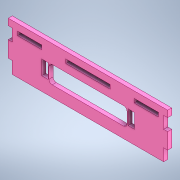
# Autodesk Inventor part: case top back
Saved by Autodesk Inventor 2022.3 (Build 263350030, 350C)
## iProperties
Created: 2021-05-28
Part Number: case top back
Material: Lead
Document SubType Name: Modeling
Designer: benka
Density: 11.34 g/cm^3
Appearance: Pink
Mass: 464.918 g
Surface Area: 220.363 cm^2
Volume: 40.9981 cm^3
Author: benka
Autodesk Inventor part; units mm, degrees
ref_plane "YZ Plane" through (0, 0, 0) normal (1, 0, 0) x (0, 1, 0)
ref_plane "XZ Plane" through (0, 0, 0) normal (0, 1, 0) x (-1, 0, 0)
ref_plane "XY Plane" through (0, 0, 0) normal (0, 0, 1) x (1, 0, 0)
sketch "Sketch1" plane through (0, 0, 0) normal (0, 0, 1) x (1, 0, 0)
  line L0 (49.9396, 9.6174) -> (57.9396, 9.6174)
  line L1 (57.9396, -8.4526) -> (49.9396, -8.4526)
  line L2 (49.9396, -8.4526) -> (49.9396, 9.6174)
  line L3 (57.9396, -8.4526) -> (57.9396, 9.6174)
  line L4 (-49.449, 9.6174) -> (-49.449, -8.4526)
  line L5 (-49.449, -8.4526) -> (-57.449, -8.4526)
  line L6 (-57.449, 9.6174) -> (-57.449, -8.4526)
  line L7 (-45.5464, 0.7392) -> (-34.5464, 0.7392)
  line L8 (-33.5464, 1.7392) -> (-33.5464, 6.2392)
  line L9 (-34.5464, 7.2392) -> (-45.5464, 7.2392)
  line L10 (-46.5464, 6.2392) -> (-46.5464, 1.7392)
  line L11 (-30.5291, -2.0275) -> (3.4709, -2.0275)
  line L12 (4.4709, -1.0275) -> (4.4709, 3.9725)
  line L13 (-31.5291, 3.9725) -> (-31.5291, -1.0275)
  circle A0 centre (-88.9996, -15.383) radius 1.5
  circle A1 centre (-64.9996, -15.383) radius 1.5
  circle A2 centre (-64.9996, 8.617) radius 1.5
  circle A3 centre (-88.9996, 8.617) radius 1.5
  arc A4 (-82.1595, 3.0543) -> (-82.1595, -9.8202) centre (-76.9996, -3.383) ccw
  arc A5 (-79.9944, -11.0702) -> (-68.8448, -4.633) centre (-76.9996, -3.383) ccw
  arc A6 (-68.8448, -2.133) -> (-79.9944, 4.3043) centre (-76.9996, -3.383) ccw
  arc A7 (-82.0034, -16.8856) -> (-62.804, -5.8009) centre (-76.9996, -3.383) ccw
  arc A8 (-63.7898, -2.133) -> (-62.804, -0.9651) centre (-63.7898, -1.133) ccw
  arc A9 (-62.804, -0.9651) -> (-82.0034, 10.1197) centre (-76.9996, -3.383) ccw
  arc A10 (-82.0034, 10.1197) -> (-82.5219, 8.682) centre (-81.6559, 9.182) ccw
  line L14 (-82.5219, 8.682) -> (-79.9944, 4.3043)
  line L15 (-82.1595, 3.0543) -> (-84.687, 7.432)
  arc A11 (-84.687, 7.432) -> (-86.1913, 7.7018) centre (-85.553, 6.932) ccw
  arc A12 (-86.1913, 7.7018) -> (-86.1913, -14.4677) centre (-76.9996, -3.383) ccw
  arc A13 (-86.1913, -14.4677) -> (-84.687, -14.1979) centre (-85.553, -13.6979) ccw
  line L16 (-84.687, -14.1979) -> (-82.1595, -9.8202)
  arc A14 (-82.5219, -15.4479) -> (-82.0034, -16.8856) centre (-81.6559, -15.9479) ccw
  line L17 (-79.9944, -11.0702) -> (-82.5219, -15.4479)
  line L18 (-63.7898, -4.633) -> (-68.8448, -4.633)
  arc A15 (-62.804, -5.8009) -> (-63.7898, -4.633) centre (-63.7898, -5.633) ccw
  line L19 (-68.8448, -2.133) -> (-63.7898, -2.133)
  circle A16 centre (64.9975, -15.3839) radius 1.5
  circle A17 centre (88.9975, -15.3839) radius 1.5
  circle A18 centre (88.9975, 8.6161) radius 1.5
  circle A19 centre (64.9975, 8.6161) radius 1.5
  line L20 (71.4751, 8.6811) -> (74.0026, 4.3033)
  arc A20 (71.9936, 10.1188) -> (71.4751, 8.6811) centre (72.3411, 9.1811) ccw
  arc A21 (91.193, -0.966) -> (71.9936, 10.1188) centre (76.9975, -3.3839) ccw
  arc A22 (85.1522, -2.1339) -> (74.0026, 4.3033) centre (76.9975, -3.3839) ccw
  line L21 (85.1522, -2.1339) -> (90.2072, -2.1339)
  arc A23 (90.2072, -2.1339) -> (91.193, -0.966) centre (90.2072, -1.1339) ccw
  arc A24 (91.193, -5.8018) -> (90.2072, -4.6339) centre (90.2072, -5.6339) ccw
  arc A25 (71.9936, -16.8866) -> (91.193, -5.8018) centre (76.9975, -3.3839) ccw
  arc A26 (74.0026, -11.0711) -> (85.1522, -4.6339) centre (76.9975, -3.3839) ccw
  line L22 (74.0026, -11.0711) -> (71.4751, -15.4489)
  line L23 (69.31, -14.1989) -> (71.8375, -9.8211)
  arc A27 (67.8057, -14.4686) -> (69.31, -14.1989) centre (68.444, -13.6989) ccw
  arc A28 (67.8057, 7.7009) -> (67.8057, -14.4686) centre (76.9975, -3.3839) ccw
  arc A29 (71.8375, 3.0533) -> (71.8375, -9.8211) centre (76.9975, -3.3839) ccw
  line L24 (71.8375, 3.0533) -> (69.31, 7.4311)
  arc A30 (69.31, 7.4311) -> (67.8057, 7.7009) centre (68.444, 6.9311) ccw
  arc A31 (71.4751, -15.4489) -> (71.9936, -16.8866) centre (72.3411, -15.9489) ccw
  line L25 (90.2072, -4.6339) -> (85.1522, -4.6339)
  line L26 (-49.449, 9.6174) -> (-57.449, 9.6174)
  line L27 (3.4709, 4.9725) -> (-30.5291, 4.9725)
  arc A32 (-34.5464, 0.7392) -> (-33.5464, 1.7392) centre (-34.5464, 1.7392) ccw
  arc A33 (-33.5464, 6.2392) -> (-34.5464, 7.2392) centre (-34.5464, 6.2392) ccw
  arc A34 (-45.5464, 7.2392) -> (-46.5464, 6.2392) centre (-45.5464, 6.2392) ccw
  arc A35 (-46.5464, 1.7392) -> (-45.5464, 0.7392) centre (-45.5464, 1.7392) ccw
  arc A36 (-31.5291, -1.0275) -> (-30.5291, -2.0275) centre (-30.5291, -1.0275) ccw
  arc A37 (-30.5291, 4.9725) -> (-31.5291, 3.9725) centre (-30.5291, 3.9725) ccw
  arc A38 (4.4709, 3.9725) -> (3.4709, 4.9725) centre (3.4709, 3.9725) ccw
  arc A39 (3.4709, -2.0275) -> (4.4709, -1.0275) centre (3.4709, -1.0275) ccw
  line L28 (-57.412, 19.6174) -> (-87.412, 19.6174) projected
  line L29 (-87.412, 19.6174) -> (-87.412, 24.6174) projected
  line L30 (-57.412, 24.6174) -> (-87.412, 24.6174) projected
  line L31 (-57.412, 19.6174) -> (-57.412, 24.6174) projected
  line L32 (27.588, 19.6174) -> (-27.412, 19.6174) projected
  line L33 (-27.412, 19.6174) -> (-27.412, 24.6174) projected
  line L34 (27.588, 24.6174) -> (-27.412, 24.6174) projected
  line L35 (27.588, 19.6174) -> (27.588, 24.6174) projected
  line L36 (87.588, 19.6174) -> (57.588, 19.6174) projected
  line L37 (57.588, 19.6174) -> (57.588, 24.6174) projected
  line L38 (87.588, 24.6174) -> (57.588, 24.6174) projected
  line L39 (87.588, 19.6174) -> (87.588, 24.6174) projected
  line L40 (94.088, -10.3826) -> (94.088, -25.3826) projected
  line L41 (99.088, -10.3826) -> (94.088, -10.3826) projected
  line L42 (99.088, 9.6181) -> (99.088, -10.3826) projected
  line L43 (99.088, 9.6181) -> (94.088, 9.6181) projected
  line L44 (94.088, 24.6181) -> (94.088, 9.6181) projected
  line L45 (99.088, 24.6181) -> (94.088, 24.6181) projected
  line L46 (99.088, 32.6174) -> (99.088, 24.6181) projected
  line L47 (-98.912, 32.6174) -> (-98.912, 24.6181) projected
  line L48 (-93.912, 24.6181) -> (-98.912, 24.6181) projected
  line L49 (-93.912, 24.6181) -> (-93.912, 9.6181) projected
  line L50 (-93.912, 9.6181) -> (-98.912, 9.6181) projected
  line L51 (-98.912, 9.6181) -> (-98.912, -10.3826) projected
  line L52 (-93.912, -10.3826) -> (-98.912, -10.3826) projected
  line L53 (-93.912, -10.3826) -> (-93.912, -25.3826) projected
  line L54 (-98.912, 32.6174) -> (99.088, 32.6174)
  line L55 (-93.912, -25.3826) -> (94.088, -25.3826)
  arc A40 (15.5314, -3.6707) -> (16.5314, -2.6707) centre (15.5314, -2.6707) ccw
  arc A41 (16.5314, 5.8293) -> (15.5314, 6.8293) centre (15.5314, 5.8293) ccw
  line L56 (5.7314, -2.6707) -> (5.7314, 5.8293)
  arc A42 (5.7314, -2.6707) -> (6.7314, -3.6707) centre (6.7314, -2.6707) ccw
  arc A43 (6.7314, 6.8293) -> (5.7314, 5.8293) centre (6.7314, 5.8293) ccw
  line L57 (6.7314, 6.8293) -> (15.5314, 6.8293)
  line L58 (6.7314, -3.6707) -> (15.5314, -3.6707)
  line L59 (23.4252, 0.4179) -> (23.4252, -9.0821)
  line L60 (37.4252, 1.4179) -> (24.4252, 1.4179)
  line L61 (24.4252, -10.0821) -> (37.4252, -10.0821)
  line L62 (38.4252, -9.0821) -> (38.4252, 0.4179)
  line L63 (16.5314, -2.6707) -> (16.5314, 5.8293)
  arc A44 (24.4252, 1.4179) -> (23.4252, 0.4179) centre (24.4252, 0.4179) ccw
  arc A45 (23.4252, -9.0821) -> (24.4252, -10.0821) centre (24.4252, -9.0821) ccw
  arc A46 (37.4252, -10.0821) -> (38.4252, -9.0821) centre (37.4252, -9.0821) ccw
  arc A47 (38.4252, 0.4179) -> (37.4252, 1.4179) centre (37.4252, 0.4179) ccw
  point P0 (-50.5662, -19.8134)
  point P1 (94.0004, -33.3808)
  point P2 (-46.5464, 0.7392)
  point P3 (-33.5464, 7.2392)
  point P4 (-33.5464, 0.7392)
  point P5 (-46.5464, 7.2392)
  point P6 (-31.5291, -2.0275)
  point P7 (4.4709, 4.9725)
  point P8 (4.4709, -2.0275)
  point P9 (-31.5291, 4.9725)
  point P10 (3.4709, -1.0275)
  point P11 (23.4252, 1.4179)
  point P12 (5.7314, -3.6707)
  point P13 (16.5314, 6.8293)
  point P14 (16.5314, -3.6707)
  point P15 (23.4252, -10.0821)
  point P16 (38.4252, -10.0821)
  point P17 (38.4252, 1.4179)
  dimension "d20" = 8
  dimension "d47" = 8
  dimension "d53" = 6.5
  dimension "d54" = 13
  dimension "d56" = 36
  dimension "d59" = 1
  dimension "d60" = 7
  dimension "d73" = 10.5
  dimension "d74" = 10.8
  dimension "d75" = 11.5
  dimension "d76" = 15
  constraints: 80 point on circle, 76 end point, 48 centre point, 32 tangent, 30 point on line, 7 equal radius, 4 horizontal, 3 perpendicular, 2 parallel, 1 collinear, 1 vertical, 1 other
  measures "d20" distance of L0.end L0.start
  measures "d47" distance of L6.start L4.start
  measures "d53" distance between parallel lines of L9 L7
  measures "d54" distance between parallel lines of L8 L10
  measures "d56" distance between parallel lines of L13 L12
  measures "d59" radius of A32
  measures "d60" distance between parallel lines of L27 L11
  measures "d73" distance between parallel lines of L57 L58
  measures "d74" distance of point (5.731, -3.671) point (16.531, -3.671)
  measures "d75" distance between parallel lines of L61 L60
  measures "d76" distance between parallel lines of L62 L59
extrude "Extrusion2" add sketch "Sketch1" along normal blind 5
sketch "Sketch2" plane through (0, 0, 0) normal (0, 0, -1) x (-1, 0, 0)
  line L0 (92.3846, -19.3253) -> (61.6146, -19.3253)
  line L1 (61.6146, -19.3253) -> (61.6146, 12.5593)
  line L2 (61.6146, 12.5593) -> (92.3846, 12.5593)
  line L3 (92.3846, 12.5593) -> (92.3846, -19.3253)
  arc A0 (82.1595, -9.8202) -> (82.1595, 3.0543) centre (76.9996, -3.383) ccw projected
  line L4 (92.3846, -19.3253) -> (61.6146, 12.5593) construction
  line L5 (61.6146, -19.3253) -> (92.3846, 12.5593) construction
  line L6 (-61.3514, -21.1002) -> (-92.6435, -21.1002)
  line L7 (-92.6435, -21.1002) -> (-92.6435, 14.3324)
  line L8 (-92.6435, 14.3324) -> (-61.3514, 14.3324)
  line L9 (-61.3514, 14.3324) -> (-61.3514, -21.1002)
  arc A1 (-67.8057, -14.4686) -> (-67.8057, 7.7009) centre (-76.9975, -3.3839) ccw projected
  line L10 (-61.3514, -21.1002) -> (-92.6435, 14.3324) construction
  line L11 (-92.6435, -21.1002) -> (-61.3514, 14.3324) construction
  point P0 (0, 0)
  constraints: 24 end point, 4 midpoint, 4 parallel, 2 horizontal, 2 perpendicular
extrude "Extrusion3" add sketch "Sketch2" against normal blind 5
sketch "Sketch3" plane through (0, 0, 0) normal (0, 0, -1) x (-1, 0, 0)
  line L0 (44.362, -11.7916) -> (-44.638, -11.7916)
  line L1 (-48.638, -7.7916) -> (-48.638, 6.2084)
  line L2 (-44.638, 10.2084) -> (44.362, 10.2084)
  line L3 (48.362, 6.2084) -> (48.362, -7.7916)
  line L4 (48.362, -11.7916) -> (-48.638, 10.2084) construction
  line L5 (-48.638, -11.7916) -> (48.362, 10.2084) construction
  arc A0 (44.362, -11.7916) -> (48.362, -7.7916) centre (44.362, -7.7916) ccw
  arc A1 (-48.638, -7.7916) -> (-44.638, -11.7916) centre (-44.638, -7.7916) ccw
  arc A2 (-44.638, 10.2084) -> (-48.638, 6.2084) centre (-44.638, 6.2084) ccw
  arc A3 (48.362, 6.2084) -> (44.362, 10.2084) centre (44.362, 6.2084) ccw
  line L6 (-99.088, -10.3826) -> (-99.088, 9.6181) projected
  line L7 (-99.088, 32.6174) -> (98.912, 32.6174) projected
  line L8 (98.912, 9.6181) -> (98.912, -10.3826) projected
  point P0 (0, 0)
  point P1 (-0.138, -0.7916)
  point P2 (-48.638, -0.7916)
  dimension "d79" = 97
  dimension "d80" = 22
  dimension "d81" = 4
  dimension "d83" = 22.409
  dimension "d84" = 50.55
  constraints: 12 end point, 8 point on circle, 8 point on line, 8 tangent, 4 centre point, 3 equal radius, 3 midpoint, 2 parallel, 1 horizontal, 1 perpendicular
  measures "d79" distance of L4.end L5.end
  measures "d80" distance of L5.start L4.end
  measures "d81" radius of A0
  measures "d83" distance between parallel lines of L7 L2
  measures "d84" distance between parallel lines of L8 L3
extrude "Extrusion4" cut sketch "Sketch3" against normal blind 5
sketch "Sketch4" plane through (0, 0, 0) normal (0, 0, -1) x (-1, 0, 0)
  arc A0 (-44.638, 10.2084) -> (-48.638, 6.2084) centre (-44.638, 6.2084) ccw projected
  line L0 (-44.638, 10.2084) -> (44.362, 10.2084) projected
  arc A1 (48.362, 6.2084) -> (44.362, 10.2084) centre (44.362, 6.2084) ccw projected
  line L1 (48.362, 6.2084) -> (48.362, -7.7916) projected
  arc A2 (44.362, -11.7916) -> (48.362, -7.7916) centre (44.362, -7.7916) ccw projected
  line L2 (44.362, -11.7916) -> (-44.638, -11.7916) projected
  arc A3 (-48.638, -7.7916) -> (-44.638, -11.7916) centre (-44.638, -7.7916) ccw projected
  line L3 (-48.638, -7.7916) -> (-48.638, 6.2084) projected
  line L4 (-94.088, 9.6181) -> (-94.088, 24.6181) projected
  line L5 (-99.088, 9.6181) -> (-94.088, 9.6181) projected
  line L6 (-99.088, -10.3826) -> (-99.088, 9.6181) projected
  line L7 (-94.088, -10.3826) -> (-99.088, -10.3826) projected
  line L8 (-94.088, -25.3826) -> (-94.088, -10.3826) projected
  line L9 (93.912, -25.3826) -> (-94.088, -25.3826) projected
  line L10 (93.912, -10.3826) -> (93.912, -25.3826) projected
  line L11 (98.912, -10.3826) -> (93.912, -10.3826) projected
  line L12 (98.912, 9.6181) -> (98.912, -10.3826) projected
  line L13 (93.912, 9.6181) -> (98.912, 9.6181) projected
  line L14 (93.912, 24.6181) -> (93.912, 9.6181) projected
  line L15 (98.912, 24.6181) -> (93.912, 24.6181) projected
  line L16 (98.912, 32.6174) -> (98.912, 24.6181) projected
  line L17 (-99.088, 32.6174) -> (98.912, 32.6174) projected
  line L18 (-99.088, 24.6181) -> (-99.088, 32.6174) projected
  line L19 (-94.088, 24.6181) -> (-99.088, 24.6181) projected
  line L20 (-87.588, 24.6174) -> (-87.588, 19.6174) projected
  line L21 (-57.588, 24.6174) -> (-87.588, 24.6174) projected
  line L22 (-57.588, 19.6174) -> (-57.588, 24.6174) projected
  line L23 (-87.588, 19.6174) -> (-57.588, 19.6174) projected
  line L24 (-27.588, 24.6174) -> (-27.588, 19.6174) projected
  line L25 (27.412, 24.6174) -> (-27.588, 24.6174) projected
  line L26 (27.412, 19.6174) -> (27.412, 24.6174) projected
  line L27 (-27.588, 19.6174) -> (27.412, 19.6174) projected
  line L28 (57.412, 24.6174) -> (57.412, 19.6174) projected
  line L29 (87.412, 24.6174) -> (57.412, 24.6174) projected
  line L30 (87.412, 19.6174) -> (87.412, 24.6174) projected
  line L31 (57.412, 19.6174) -> (87.412, 19.6174) projected
  line L32 (57.449, 9.6174) -> (49.449, 9.6174) projected
  line L33 (57.449, -8.4526) -> (57.449, 9.6174) projected
  line L34 (49.449, -8.4526) -> (57.449, -8.4526) projected
  line L35 (49.449, 9.6174) -> (49.449, -8.4526) projected
  line L36 (-57.9396, -8.4526) -> (-49.9396, -8.4526) projected
  line L37 (-57.9396, 9.6174) -> (-57.9396, -8.4526) projected
  line L38 (-49.9396, 9.6174) -> (-57.9396, 9.6174) projected
  line L39 (-49.9396, -8.4526) -> (-49.9396, 9.6174) projected
  point P0 (0, 0)
body "Solid2"
